Autodesk Inventor part; units mm, degrees
(part 2 of 2)
sketch "スケッチ16" plane through (250, 25, 10) normal (0, 1, 0) x (1, 0, 0)
  line L0 (-250, 20) -> (-250, 0) projected
  line L1 (-250, 0) -> (0, 0) projected
  line L2 (0, 0) -> (0, 20) projected
  line L3 (-250, 20) -> (0, 20) projected
  line L4 (-175, 16) -> (-158.2685, 16) projected
  line L5 (-158.2685, 16) -> (-175, 6.3111) projected
  line L6 (-175, 6.3111) -> (-175, 16) projected
  line L7 (-104, 13.8495) -> (-104, 4) projected
  line L8 (-104, 4) -> (-121.0089, 4) projected
  line L9 (-121.0089, 4) -> (-104, 13.8495) projected
  line L10 (-83, 16) -> (-72.9486, 16) projected
  line L11 (-72.9486, 16) -> (-83, 6.7218) projected
  line L12 (-83, 6.7218) -> (-83, 16) projected
  line L13 (-50, 16) -> (-43.9509, 16) projected
  line L14 (-43.9509, 16) -> (-50, 7.4601) projected
  line L15 (-50, 7.4601) -> (-50, 16) projected
  line L16 (-25, 16) -> (-18.9509, 16) projected
  line L17 (-18.9509, 16) -> (-25, 7.4601) projected
  line L18 (-25, 7.4601) -> (-25, 16) projected
  line L19 (-4, 4) -> (-10.0491, 4) projected
  line L20 (-10.0491, 4) -> (-4, 12.5399) projected
  line L21 (-4, 12.5399) -> (-4, 4) projected
  line L22 (-35.0491, 4) -> (-29, 12.5399) projected
  line L23 (-29, 12.5399) -> (-29, 4) projected
  line L24 (-29, 4) -> (-35.0491, 4) projected
  line L25 (-54, 4) -> (-63.1716, 4) projected
  line L26 (-63.1716, 4) -> (-54, 13.1716) projected
  line L27 (-54, 13.1716) -> (-54, 4) projected
  line L28 (-87, 4) -> (-97.0514, 4) projected
  line L29 (-97.0514, 4) -> (-87, 13.2782) projected
  line L30 (-87, 13.2782) -> (-87, 4) projected
  line L31 (-133.0311, 16) -> (-150, 6.3035) projected
  line L32 (-150, 6.3035) -> (-150, 16) projected
  line L33 (-150, 16) -> (-133.0311, 16) projected
  line L34 (-200, 16) -> (-183.0311, 16) projected
  line L35 (-183.0311, 16) -> (-200, 6.3035) projected
  line L36 (-200, 6.3035) -> (-200, 16) projected
  line L37 (-204, 4) -> (-240.5948, 4) projected
  line L38 (-240.5948, 4) -> (-204, 14.2649) projected
  line L39 (-204, 14.2649) -> (-204, 4) projected
  line L40 (-154, 13.8495) -> (-154, 4) projected
  line L41 (-154, 4) -> (-171.0089, 4) projected
  line L42 (-171.0089, 4) -> (-154, 13.8495) projected
  line L43 (-108.2685, 16) -> (-125, 6.3111) projected
  line L44 (-125, 6.3111) -> (-125, 16) projected
  line L45 (-125, 16) -> (-108.2685, 16) projected
  line L46 (-70, 4) -> (-80.0514, 4) projected
  line L47 (-80.0514, 4) -> (-70, 13.2782) projected
  line L48 (-70, 13.2782) -> (-70, 4) projected
  line L49 (-47.5491, 4) -> (-41.5, 12.5399) projected
  line L50 (-41.5, 12.5399) -> (-41.5, 4) projected
  line L51 (-41.5, 4) -> (-47.5491, 4) projected
  line L52 (-16.5, 4) -> (-22.5491, 4) projected
  line L53 (-22.5491, 4) -> (-16.5, 12.5399) projected
  line L54 (-16.5, 12.5399) -> (-16.5, 4) projected
  line L55 (-12.5, 16) -> (-6.4509, 16) projected
  line L56 (-6.4509, 16) -> (-12.5, 7.4601) projected
  line L57 (-12.5, 7.4601) -> (-12.5, 16) projected
  line L58 (-37.5, 16) -> (-31.4509, 16) projected
  line L59 (-31.4509, 16) -> (-37.5, 7.4601) projected
  line L60 (-37.5, 7.4601) -> (-37.5, 16) projected
  line L61 (-66, 16) -> (-56.8284, 16) projected
  line L62 (-56.8284, 16) -> (-66, 6.8284) projected
  line L63 (-66, 6.8284) -> (-66, 16) projected
  line L64 (-100, 16) -> (-89.9486, 16) projected
  line L65 (-89.9486, 16) -> (-100, 6.7218) projected
  line L66 (-100, 6.7218) -> (-100, 16) projected
  line L67 (-145.9689, 4) -> (-129, 13.6965) projected
  line L68 (-129, 13.6965) -> (-129, 4) projected
  line L69 (-129, 4) -> (-145.9689, 4) projected
  line L70 (-179, 13.6965) -> (-179, 4) projected
  line L71 (-179, 4) -> (-195.9689, 4) projected
  line L72 (-195.9689, 4) -> (-179, 13.6965) projected
  line L73 (-248, 16) -> (-211.4052, 16) projected
  line L74 (-211.4052, 16) -> (-248, 6.0772) projected
  line L75 (-248, 6.0772) -> (-248, 16) projected
  point P0 (-250, 10)
extrude "押し出し25" add sketch "スケッチ16" against normal blind 4 contours L13 L14 L15 | L25 L26 L27 | L49 L50 L51 | L61 L62 L63
extrude "押し出し26" cut sketch "スケッチ15" against normal blind 4 contours L11 L54 L109 L2 | L6 L41 L5 | L110 L104 L89 L14 | L12 L109 L54 | L41 L20 L19 L24 L5 | L89 L90 L15 L14 | L25 L7 L10 L9
sketch "スケッチ17" plane through (250, -25, -10) normal (0, -1, 0) x (1, 0, 0)
  line L0 (-31.0405, 4) -> (-25, 4) projected
  line L1 (-248, 13.9228) -> (-211.4052, 4) projected
  line L2 (-211.4052, 4) -> (-248, 4) projected
  line L3 (-248, 4) -> (-248, 13.9228) projected
  line L4 (-179, 16) -> (-179, 6.3035) projected
  line L5 (-179, 6.3035) -> (-195.9689, 16) projected
  line L6 (-195.9689, 16) -> (-179, 16) projected
  line L7 (-129, 6.3035) -> (-145.9689, 16) projected
  line L8 (-145.9689, 16) -> (-129, 16) projected
  line L9 (-129, 16) -> (-129, 6.3035) projected
  line L10 (-89.9486, 4) -> (-100, 4) projected
  line L11 (-100, 4) -> (-100, 13.2782) projected
  line L12 (-100, 13.2782) -> (-89.9486, 4) projected
  line L13 (-56.8284, 4) -> (-66, 4) projected
  line L14 (-66, 4) -> (-66, 13.1716) projected
  line L15 (-66, 13.1716) -> (-56.8284, 4) projected
  line L16 (-31.4509, 4) -> (-37.5, 4) projected
  line L17 (-37.5, 4) -> (-37.5, 12.5399) projected
  line L18 (-37.5, 12.5399) -> (-31.4509, 4) projected
  line L19 (-6.4509, 4) -> (-12.5, 4) projected
  line L20 (-12.5, 4) -> (-12.5, 12.5399) projected
  line L21 (-12.5, 12.5399) -> (-6.4509, 4) projected
  line L22 (-22.5491, 16) -> (-16.5, 16) projected
  line L23 (-16.5, 16) -> (-16.5, 7.4601) projected
  line L24 (-16.5, 7.4601) -> (-22.5491, 16) projected
  line L25 (-41.5, 7.4601) -> (-47.5491, 16) projected
  line L26 (-47.5491, 16) -> (-41.5, 16) projected
  line L27 (-41.5, 16) -> (-41.5, 7.4601) projected
  line L28 (-80.0514, 16) -> (-70, 16) projected
  line L29 (-70, 16) -> (-70, 6.7218) projected
  line L30 (-70, 6.7218) -> (-80.0514, 16) projected
  line L31 (-125, 13.6889) -> (-108.2685, 4) projected
  line L32 (-108.2685, 4) -> (-125, 4) projected
  line L33 (-125, 4) -> (-125, 13.6889) projected
  line L34 (-154, 16) -> (-154, 6.1505) projected
  line L35 (-154, 6.1505) -> (-171.0089, 16) projected
  line L36 (-171.0089, 16) -> (-154, 16) projected
  line L37 (-240.5948, 16) -> (-204, 16) projected
  line L38 (-204, 16) -> (-204, 5.7351) projected
  line L39 (-204, 5.7351) -> (-240.5948, 16) projected
  line L40 (-183.0311, 4) -> (-200, 4) projected
  line L41 (-200, 4) -> (-200, 13.6965) projected
  line L42 (-200, 13.6965) -> (-183.0311, 4) projected
  line L43 (-150, 13.6965) -> (-133.0311, 4) projected
  line L44 (-133.0311, 4) -> (-150, 4) projected
  line L45 (-150, 4) -> (-150, 13.6965) projected
  line L46 (-97.0514, 16) -> (-87, 16) projected
  line L47 (-87, 16) -> (-87, 6.7218) projected
  line L48 (-87, 6.7218) -> (-97.0514, 16) projected
  line L49 (-63.1716, 16) -> (-54, 16) projected
  line L50 (-54, 16) -> (-54, 6.8284) projected
  line L51 (-54, 6.8284) -> (-63.1716, 16) projected
  line L52 (-29, 7.4601) -> (-35.0491, 16) projected
  line L53 (-35.0491, 16) -> (-29, 16) projected
  line L54 (-29, 16) -> (-29, 7.4601) projected
  line L55 (-10.0491, 16) -> (-4, 16) projected
  line L56 (-4, 16) -> (-4, 7.4601) projected
  line L57 (-4, 7.4601) -> (-10.0491, 16) projected
  line L58 (-18.9509, 4) -> (-25, 4) projected
  line L59 (-25, 4) -> (-25, 12.5399) projected
  line L60 (-25, 12.5399) -> (-18.9509, 4) projected
  line L61 (-43.9509, 4) -> (-50, 4) projected
  line L62 (-50, 4) -> (-50, 12.5399) projected
  line L63 (-50, 12.5399) -> (-43.9509, 4) projected
  line L64 (-72.9486, 4) -> (-83, 4) projected
  line L65 (-83, 4) -> (-83, 13.2782) projected
  line L66 (-83, 13.2782) -> (-72.9486, 4) projected
  line L67 (-104, 16) -> (-104, 6.1505) projected
  line L68 (-104, 6.1505) -> (-121.0089, 16) projected
  line L69 (-121.0089, 16) -> (-104, 16) projected
  line L70 (-158.2685, 4) -> (-175, 4) projected
  line L71 (-175, 4) -> (-175, 13.6889) projected
  line L72 (-175, 13.6889) -> (-158.2685, 4) projected
  line L73 (-250, 20) -> (-250, 0) projected
  line L74 (-250, 0) -> (0, 0) projected
  line L75 (0, 0) -> (0, 20) projected
  line L76 (0, 20) -> (-250, 20) projected
  point P0 (-250, 10)
extrude "押し出し27" add sketch "スケッチ17" against normal blind 4 contours L13 L14 L15 | L25 L26 L27 | L49 L50 L51 | L61 L62 L63
mirror "ミラー4" about plane through (0, 0, 0) normal (0, 1, 0) of "押し出し26"
sketch "スケッチ18" plane through (250, -25, -10) normal (0, 0, -1) x (-1, 0, 0)
  line L0 (4, 46) -> (4, 50) projected
  line L1 (62.6667, 4) -> (50, 4) projected
  line L2 (4, 46) -> (52.1102, 46)
  line L3 (52.1102, 46) -> (52.1102, 4)
  line L4 (52.1102, 4) -> (4, 4)
  line L5 (4, 4) -> (4, 46)
  line L6 (53.3333, 4) -> (66, 4) projected
  line L7 (4, 46) -> (54, 46)
  line L8 (54, 46) -> (54, 4)
  line L9 (54, 4) -> (4, 4)
  line L10 (4, 4) -> (4, 46)
  point P0 (250, 25)
  dimension "d290" = 50
  constraints: 16 end point, 4 parallel, 2 horizontal, 2 perpendicular, 2 point on line
  measures "d290" distance of L8.end L9.end
extrude "押し出し28" add sketch "スケッチ18" against normal blind 4 contours L1 L4 L5 L2 L3
sketch "スケッチ19" plane through (250, -25, 10) normal (0, 0, 1) x (1, 0, 0)
  line L0 (-4, 4) -> (0, 4) projected
  line L1 (-50, 46) -> (-47.9595, 46) projected
  line L2 (-4, 4) -> (-47.9595, 4)
  line L3 (-47.9595, 4) -> (-47.9595, 46)
  line L4 (-47.9595, 46) -> (-4, 46)
  line L5 (-4, 46) -> (-4, 4)
  line L6 (-4, 4) -> (-54, 4)
  line L7 (-54, 4) -> (-54, 46)
  line L8 (-54, 46) -> (-4, 46)
  line L9 (-4, 46) -> (-4, 4)
  point P0 (-250, 25)
  dimension "d293" = 50
  dimension "d294" = 42
  constraints: 16 end point, 4 parallel, 2 horizontal, 2 perpendicular
  measures "d293" distance of L7.end L8.end
  measures "d294" distance of L6.end L7.end
extrude "押し出し29" add sketch "スケッチ19" against normal blind 4
sketch "スケッチ20" plane through (250, -25, -10) normal (0, 0, -1) x (-1, 0, 0)
  point P0 (250, 25)
extrude "押し出し30" add sketch "SCBottom" against normal blind 4 contours L99 L90 L43 L49 | L49 L43 L90 L101
sketch "スケッチ21" plane through (250, -25, 10) normal (0, 0, 1) x (1, 0, 0)
  line L0 (-54, 11.2801) -> (-57.92, 25) projected
  line L1 (-57.92, 25) -> (-54, 38.7199) projected
  line L2 (-54, 38.7199) -> (-54, 11.2801) projected
  line L3 (-250, 50) -> (-250, 0) projected
  line L4 (0, 0) -> (-250, 0) projected
  line L5 (0, 0) -> (0, 50) projected
  line L6 (-250, 50) -> (0, 50) projected
  line L7 (-248, 6.7649) -> (-248, 43.1716) projected
  line L8 (-248, 43.1716) -> (-229.3733, 24.5449) projected
  line L9 (-229.3733, 24.5449) -> (-248, 6.7649) projected
  line L10 (-197.7639, 46) -> (-181.2361, 46) projected
  line L11 (-181.2361, 46) -> (-189.5, 29.4721) projected
  line L12 (-189.5, 29.4721) -> (-197.7639, 46) projected
  line L13 (-162.2639, 25) -> (-154, 41.5279) projected
  line L14 (-154, 41.5279) -> (-154, 8.4721) projected
  line L15 (-154, 8.4721) -> (-162.2639, 25) projected
  line L16 (-129, 8.4721) -> (-137.2639, 25) projected
  line L17 (-137.2639, 25) -> (-129, 41.5279) projected
  line L18 (-129, 41.5279) -> (-129, 8.4721) projected
  line L19 (-104, 8.4721) -> (-112.2639, 25) projected
  line L20 (-112.2639, 25) -> (-104, 41.5279) projected
  line L21 (-104, 41.5279) -> (-104, 8.4721) projected
  line L22 (-87, 10.764) -> (-91.4064, 25) projected
  line L23 (-91.4064, 25) -> (-87, 39.236) projected
  line L24 (-87, 39.236) -> (-87, 10.764) projected
  line L25 (-74.4064, 25) -> (-70, 39.236) projected
  line L26 (-70, 39.236) -> (-70, 10.764) projected
  line L27 (-70, 10.764) -> (-74.4064, 25) projected
  line L28 (-63.92, 46) -> (-56.08, 46) projected
  line L29 (-56.08, 46) -> (-60, 32.2801) projected
  line L30 (-60, 32.2801) -> (-63.92, 46) projected
  line L31 (-72.0936, 4) -> (-80.9064, 4) projected
  line L32 (-80.9064, 4) -> (-76.5, 18.236) projected
  line L33 (-76.5, 18.236) -> (-72.0936, 4) projected
  line L34 (-89.0936, 4) -> (-97.9064, 4) projected
  line L35 (-97.9064, 4) -> (-93.5, 18.236) projected
  line L36 (-93.5, 18.236) -> (-89.0936, 4) projected
  line L37 (-122.7639, 46) -> (-106.2361, 46) projected
  line L38 (-106.2361, 46) -> (-114.5, 29.4721) projected
  line L39 (-114.5, 29.4721) -> (-122.7639, 46) projected
  line L40 (-131.2361, 4) -> (-147.7639, 4) projected
  line L41 (-147.7639, 4) -> (-139.5, 20.5279) projected
  line L42 (-139.5, 20.5279) -> (-131.2361, 4) projected
  line L43 (-156.2361, 4) -> (-172.7639, 4) projected
  line L44 (-172.7639, 4) -> (-164.5, 20.5279) projected
  line L45 (-164.5, 20.5279) -> (-156.2361, 4) projected
  line L46 (-187.2639, 25) -> (-179, 41.5279) projected
  line L47 (-179, 41.5279) -> (-179, 8.4721) projected
  line L48 (-179, 8.4721) -> (-187.2639, 25) projected
  line L49 (-191.7361, 25) -> (-200, 8.4721) projected
  line L50 (-200, 8.4721) -> (-200, 41.5279) projected
  line L51 (-200, 41.5279) -> (-191.7361, 25) projected
  line L52 (-172.7639, 46) -> (-156.2361, 46) projected
  line L53 (-156.2361, 46) -> (-164.5, 29.4721) projected
  line L54 (-164.5, 29.4721) -> (-172.7639, 46) projected
  line L55 (-150, 41.5279) -> (-141.7361, 25) projected
  line L56 (-141.7361, 25) -> (-150, 8.4721) projected
  line L57 (-150, 8.4721) -> (-150, 41.5279) projected
  line L58 (-106.2361, 4) -> (-122.7639, 4) projected
  line L59 (-122.7639, 4) -> (-114.5, 20.5279) projected
  line L60 (-114.5, 20.5279) -> (-106.2361, 4) projected
  line L61 (-97.9064, 46) -> (-89.0936, 46) projected
  line L62 (-89.0936, 46) -> (-93.5, 31.764) projected
  line L63 (-93.5, 31.764) -> (-97.9064, 46) projected
  line L64 (-80.9064, 46) -> (-72.0936, 46) projected
  line L65 (-72.0936, 46) -> (-76.5, 31.764) projected
  line L66 (-76.5, 31.764) -> (-80.9064, 46) projected
  line L67 (-56.08, 4) -> (-63.92, 4) projected
  line L68 (-63.92, 4) -> (-60, 17.7199) projected
  line L69 (-60, 17.7199) -> (-56.08, 4) projected
  line L70 (-62.08, 25) -> (-66, 11.2801) projected
  line L71 (-66, 11.2801) -> (-66, 38.7199) projected
  line L72 (-66, 38.7199) -> (-62.08, 25) projected
  line L73 (-78.5936, 25) -> (-83, 10.764) projected
  line L74 (-83, 10.764) -> (-83, 39.236) projected
  line L75 (-83, 39.236) -> (-78.5936, 25) projected
  line L76 (-95.5936, 25) -> (-100, 10.764) projected
  line L77 (-100, 10.764) -> (-100, 39.236) projected
  line L78 (-100, 39.236) -> (-95.5936, 25) projected
  line L79 (-125, 41.5279) -> (-116.7361, 25) projected
  line L80 (-116.7361, 25) -> (-125, 8.4721) projected
  line L81 (-125, 8.4721) -> (-125, 41.5279) projected
  line L82 (-147.7639, 46) -> (-131.2361, 46) projected
  line L83 (-131.2361, 46) -> (-139.5, 29.4721) projected
  line L84 (-139.5, 29.4721) -> (-147.7639, 46) projected
  line L85 (-166.7361, 25) -> (-175, 8.4721) projected
  line L86 (-175, 8.4721) -> (-175, 41.5279) projected
  line L87 (-175, 41.5279) -> (-166.7361, 25) projected
  line L88 (-197.7639, 4) -> (-189.5, 20.5279) projected
  line L89 (-189.5, 20.5279) -> (-181.2361, 4) projected
  line L90 (-181.2361, 4) -> (-197.7639, 4) projected
  line L91 (-226.4791, 27.3075) -> (-245.1716, 46) projected
  line L92 (-245.1716, 46) -> (-206.8966, 46) projected
  line L93 (-206.8966, 46) -> (-226.4791, 27.3075) projected
  line L94 (-245.1034, 4) -> (-226.5441, 21.7157) projected
  line L95 (-226.5441, 21.7157) -> (-208.8284, 4) projected
  line L96 (-208.8284, 4) -> (-245.1034, 4) projected
  line L97 (-204, 43.2351) -> (-204, 4.8284) projected
  line L98 (-204, 4.8284) -> (-223.6499, 24.4784) projected
  line L99 (-223.6499, 24.4784) -> (-204, 43.2351) projected
  point P0 (-250, 25)
extrude "押し出し31" add sketch "スケッチ21" against normal blind 4 contours L0 L1 L2
sketch "スケッチ22" plane through (250, -25, 10) normal (0, 0, 1) x (1, 0, 0)
  line L0 (-250, 50) -> (-250, 0) projected
  line L1 (0, 0) -> (-250, 0) projected
  line L2 (0, 0) -> (0, 50) projected
  line L3 (-250, 50) -> (0, 50) projected
  line L4 (-248, 6.7649) -> (-248, 43.1716) projected
  line L5 (-248, 43.1716) -> (-229.3733, 24.5449) projected
  line L6 (-229.3733, 24.5449) -> (-248, 6.7649) projected
  line L7 (-197.7639, 46) -> (-181.2361, 46) projected
  line L8 (-181.2361, 46) -> (-189.5, 29.4721) projected
  line L9 (-189.5, 29.4721) -> (-197.7639, 46) projected
  line L10 (-162.2639, 25) -> (-154, 41.5279) projected
  line L11 (-154, 41.5279) -> (-154, 8.4721) projected
  line L12 (-154, 8.4721) -> (-162.2639, 25) projected
  line L13 (-129, 8.4721) -> (-137.2639, 25) projected
  line L14 (-137.2639, 25) -> (-129, 41.5279) projected
  line L15 (-129, 41.5279) -> (-129, 8.4721) projected
  line L16 (-104, 8.4721) -> (-112.2639, 25) projected
  line L17 (-112.2639, 25) -> (-104, 41.5279) projected
  line L18 (-104, 41.5279) -> (-104, 8.4721) projected
  line L19 (-87, 10.764) -> (-91.4064, 25) projected
  line L20 (-91.4064, 25) -> (-87, 39.236) projected
  line L21 (-87, 39.236) -> (-87, 10.764) projected
  line L22 (-74.4064, 25) -> (-70, 39.236) projected
  line L23 (-70, 39.236) -> (-70, 10.764) projected
  line L24 (-70, 10.764) -> (-74.4064, 25) projected
  line L25 (-63.92, 46) -> (-56.08, 46) projected
  line L26 (-56.08, 46) -> (-60, 32.2801) projected
  line L27 (-60, 32.2801) -> (-63.92, 46) projected
  line L28 (-72.0936, 4) -> (-80.9064, 4) projected
  line L29 (-80.9064, 4) -> (-76.5, 18.236) projected
  line L30 (-76.5, 18.236) -> (-72.0936, 4) projected
  line L31 (-89.0936, 4) -> (-97.9064, 4) projected
  line L32 (-97.9064, 4) -> (-93.5, 18.236) projected
  line L33 (-93.5, 18.236) -> (-89.0936, 4) projected
  line L34 (-122.7639, 46) -> (-106.2361, 46) projected
  line L35 (-106.2361, 46) -> (-114.5, 29.4721) projected
  line L36 (-114.5, 29.4721) -> (-122.7639, 46) projected
  line L37 (-131.2361, 4) -> (-147.7639, 4) projected
  line L38 (-147.7639, 4) -> (-139.5, 20.5279) projected
  line L39 (-139.5, 20.5279) -> (-131.2361, 4) projected
  line L40 (-156.2361, 4) -> (-172.7639, 4) projected
  line L41 (-172.7639, 4) -> (-164.5, 20.5279) projected
  line L42 (-164.5, 20.5279) -> (-156.2361, 4) projected
  line L43 (-187.2639, 25) -> (-179, 41.5279) projected
  line L44 (-179, 41.5279) -> (-179, 8.4721) projected
  line L45 (-179, 8.4721) -> (-187.2639, 25) projected
  line L46 (-191.7361, 25) -> (-200, 8.4721) projected
  line L47 (-200, 8.4721) -> (-200, 41.5279) projected
  line L48 (-200, 41.5279) -> (-191.7361, 25) projected
  line L49 (-172.7639, 46) -> (-156.2361, 46) projected
  line L50 (-156.2361, 46) -> (-164.5, 29.4721) projected
  line L51 (-164.5, 29.4721) -> (-172.7639, 46) projected
  line L52 (-150, 41.5279) -> (-141.7361, 25) projected
  line L53 (-141.7361, 25) -> (-150, 8.4721) projected
  line L54 (-150, 8.4721) -> (-150, 41.5279) projected
  line L55 (-106.2361, 4) -> (-122.7639, 4) projected
  line L56 (-122.7639, 4) -> (-114.5, 20.5279) projected
  line L57 (-114.5, 20.5279) -> (-106.2361, 4) projected
  line L58 (-97.9064, 46) -> (-89.0936, 46) projected
  line L59 (-89.0936, 46) -> (-93.5, 31.764) projected
  line L60 (-93.5, 31.764) -> (-97.9064, 46) projected
  line L61 (-80.9064, 46) -> (-72.0936, 46) projected
  line L62 (-72.0936, 46) -> (-76.5, 31.764) projected
  line L63 (-76.5, 31.764) -> (-80.9064, 46) projected
  line L64 (-56.08, 4) -> (-63.92, 4) projected
  line L65 (-63.92, 4) -> (-60, 17.7199) projected
  line L66 (-60, 17.7199) -> (-56.08, 4) projected
  line L67 (-62.08, 25) -> (-66, 11.2801) projected
  line L68 (-66, 11.2801) -> (-66, 38.7199) projected
  line L69 (-66, 38.7199) -> (-62.08, 25) projected
  line L70 (-78.5936, 25) -> (-83, 10.764) projected
  line L71 (-83, 10.764) -> (-83, 39.236) projected
  line L72 (-83, 39.236) -> (-78.5936, 25) projected
  line L73 (-95.5936, 25) -> (-100, 10.764) projected
  line L74 (-100, 10.764) -> (-100, 39.236) projected
  line L75 (-100, 39.236) -> (-95.5936, 25) projected
  line L76 (-125, 41.5279) -> (-116.7361, 25) projected
  line L77 (-116.7361, 25) -> (-125, 8.4721) projected
  line L78 (-125, 8.4721) -> (-125, 41.5279) projected
  line L79 (-147.7639, 46) -> (-131.2361, 46) projected
  line L80 (-131.2361, 46) -> (-139.5, 29.4721) projected
  line L81 (-139.5, 29.4721) -> (-147.7639, 46) projected
  line L82 (-166.7361, 25) -> (-175, 8.4721) projected
  line L83 (-175, 8.4721) -> (-175, 41.5279) projected
  line L84 (-175, 41.5279) -> (-166.7361, 25) projected
  line L85 (-197.7639, 4) -> (-189.5, 20.5279) projected
  line L86 (-189.5, 20.5279) -> (-181.2361, 4) projected
  line L87 (-181.2361, 4) -> (-197.7639, 4) projected
  line L88 (-226.4791, 27.3075) -> (-245.1716, 46) projected
  line L89 (-245.1716, 46) -> (-206.8966, 46) projected
  line L90 (-206.8966, 46) -> (-226.4791, 27.3075) projected
  line L91 (-245.1034, 4) -> (-226.5441, 21.7157) projected
  line L92 (-226.5441, 21.7157) -> (-208.8284, 4) projected
  line L93 (-208.8284, 4) -> (-245.1034, 4) projected
  line L94 (-204, 43.2351) -> (-204, 4.8284) projected
  line L95 (-204, 4.8284) -> (-223.6499, 24.4784) projected
  line L96 (-223.6499, 24.4784) -> (-204, 43.2351) projected
  line L97 (-58.279, 25) -> (-48.0006, 4)
  line L98 (-50, 4) -> (-43.864, 4) projected
  line L99 (-58.279, 25) -> (-48.0006, 46)
  line L100 (-50, 46) -> (-43.864, 46) projected
  line L101 (-63.92, 46) -> (-60, 32.2801) projected
  line L102 (-60, 32.2801) -> (-53.2848, 46)
  line L103 (-53.3333, 46) -> (-46, 46) projected
  line L104 (-50, 4) -> (-46, 4)
  line L105 (-46, 4) -> (-46, 46)
  line L106 (-46, 46) -> (-50, 46)
  line L107 (-50, 46) -> (-50, 4)
  line L108 (-3.6692, 25) -> (16.3308, 25)
  line L109 (0, 46) -> (0, 4) projected
  line L110 (-3.6692, 25) -> (16.3308, 25) construction
  line L111 (-16.5, 4) -> (-10.0491, 4) projected
  line L112 (-15.3736, 4) -> (-19.3736, 4)
  line L113 (-19.3736, 4) -> (-19.3736, 46)
  line L114 (-19.3736, 46) -> (-15.3736, 46)
  line L115 (-15.3736, 46) -> (-15.3736, 4)
  line L116 (-30.6182, 3.9696) -> (-34.6182, 3.9696)
  line L117 (-34.6182, 3.9696) -> (-34.6182, 45.9696)
  line L118 (-34.6182, 45.9696) -> (-30.6182, 45.9696)
  line L119 (-30.6182, 45.9696) -> (-30.6182, 3.9696)
  line L120 (-4, 4) -> (0, 4) projected
  line L121 (-4, 4) -> (-15.3736, 46)
  line L122 (-30.6182, 45.9696) -> (-19.3736, 4)
  line L123 (-34.6182, 3.9696) -> (-46, 46)
  line L124 (-36.5487, 3.4469) -> (-47.9305, 45.4772)
  line L125 (-34.6182, 11.6212) -> (-44.0695, 46.5228)
  line L126 (-32.5501, 45.4521) -> (-21.3054, 3.4824)
  line L127 (-15.3736, 38.3484) -> (-6.0638, 3.9696)
  line L128 (-5.5304, 2) -> (0, 2)
  line L129 (-13.3015, 46) -> (-2.4696, 6)
  line L130 (-2.4696, 6) -> (0, 6)
  line L131 (-28.6863, 46.4872) -> (-19.3736, 11.7281)
  line L132 (-250, 50) -> (-250, 0) projected
  line L133 (0, 0) -> (-250, 0) projected
  line L134 (0, 0) -> (0, 50) projected
  line L135 (-250, 50) -> (0, 50) projected
  line L136 (-248, 6.7649) -> (-248, 43.1716) projected
  line L137 (-248, 43.1716) -> (-229.3733, 24.5449) projected
  line L138 (-229.3733, 24.5449) -> (-248, 6.7649) projected
  line L139 (-197.7639, 46) -> (-181.2361, 46) projected
  line L140 (-181.2361, 46) -> (-189.5, 29.4721) projected
  line L141 (-189.5, 29.4721) -> (-197.7639, 46) projected
  line L142 (-162.2639, 25) -> (-154, 41.5279) projected
  line L143 (-154, 41.5279) -> (-154, 8.4721) projected
  line L144 (-154, 8.4721) -> (-162.2639, 25) projected
  line L145 (-129, 8.4721) -> (-137.2639, 25) projected
  line L146 (-137.2639, 25) -> (-129, 41.5279) projected
  line L147 (-129, 41.5279) -> (-129, 8.4721) projected
  line L148 (-104, 8.4721) -> (-112.2639, 25) projected
  line L149 (-112.2639, 25) -> (-104, 41.5279) projected
  line L150 (-104, 41.5279) -> (-104, 8.4721) projected
  line L151 (-87, 10.764) -> (-91.4064, 25) projected
  line L152 (-91.4064, 25) -> (-87, 39.236) projected
  line L153 (-87, 39.236) -> (-87, 10.764) projected
  line L154 (-74.4064, 25) -> (-70, 39.236) projected
  line L155 (-70, 39.236) -> (-70, 10.764) projected
  line L156 (-70, 10.764) -> (-74.4064, 25) projected
  line L157 (-63.92, 46) -> (-56.08, 46) projected
  line L158 (-56.08, 46) -> (-60, 32.2801) projected
  line L159 (-60, 32.2801) -> (-63.92, 46) projected
  line L160 (-72.0936, 4) -> (-80.9064, 4) projected
  line L161 (-80.9064, 4) -> (-76.5, 18.236) projected
  line L162 (-76.5, 18.236) -> (-72.0936, 4) projected
  line L163 (-89.0936, 4) -> (-97.9064, 4) projected
  line L164 (-97.9064, 4) -> (-93.5, 18.236) projected
  line L165 (-93.5, 18.236) -> (-89.0936, 4) projected
  line L166 (-122.7639, 46) -> (-106.2361, 46) projected
  line L167 (-106.2361, 46) -> (-114.5, 29.4721) projected
  line L168 (-114.5, 29.4721) -> (-122.7639, 46) projected
  line L169 (-131.2361, 4) -> (-147.7639, 4) projected
  line L170 (-147.7639, 4) -> (-139.5, 20.5279) projected
  line L171 (-139.5, 20.5279) -> (-131.2361, 4) projected
  line L172 (-156.2361, 4) -> (-172.7639, 4) projected
  line L173 (-172.7639, 4) -> (-164.5, 20.5279) projected
  line L174 (-164.5, 20.5279) -> (-156.2361, 4) projected
  line L175 (-187.2639, 25) -> (-179, 41.5279) projected
  line L176 (-179, 41.5279) -> (-179, 8.4721) projected
  line L177 (-179, 8.4721) -> (-187.2639, 25) projected
  line L178 (-191.7361, 25) -> (-200, 8.4721) projected
  line L179 (-200, 8.4721) -> (-200, 41.5279) projected
  line L180 (-200, 41.5279) -> (-191.7361, 25) projected
  line L181 (-172.7639, 46) -> (-156.2361, 46) projected
  line L182 (-156.2361, 46) -> (-164.5, 29.4721) projected
  line L183 (-164.5, 29.4721) -> (-172.7639, 46) projected
  line L184 (-150, 41.5279) -> (-141.7361, 25) projected
  line L185 (-141.7361, 25) -> (-150, 8.4721) projected
  line L186 (-150, 8.4721) -> (-150, 41.5279) projected
  line L187 (-106.2361, 4) -> (-122.7639, 4) projected
  line L188 (-122.7639, 4) -> (-114.5, 20.5279) projected
  line L189 (-114.5, 20.5279) -> (-106.2361, 4) projected
  line L190 (-97.9064, 46) -> (-89.0936, 46) projected
  line L191 (-89.0936, 46) -> (-93.5, 31.764) projected
  line L192 (-93.5, 31.764) -> (-97.9064, 46) projected
  line L193 (-80.9064, 46) -> (-72.0936, 46) projected
  line L194 (-72.0936, 46) -> (-76.5, 31.764) projected
  line L195 (-76.5, 31.764) -> (-80.9064, 46) projected
  line L196 (-56.08, 4) -> (-63.92, 4) projected
  line L197 (-63.92, 4) -> (-60, 17.7199) projected
  line L198 (-60, 17.7199) -> (-56.08, 4) projected
  line L199 (-62.08, 25) -> (-66, 11.2801) projected
  line L200 (-66, 11.2801) -> (-66, 38.7199) projected
  line L201 (-66, 38.7199) -> (-62.08, 25) projected
  line L202 (-78.5936, 25) -> (-83, 10.764) projected
  line L203 (-83, 10.764) -> (-83, 39.236) projected
  line L204 (-83, 39.236) -> (-78.5936, 25) projected
  line L205 (-95.5936, 25) -> (-100, 10.764) projected
  line L206 (-100, 10.764) -> (-100, 39.236) projected
  line L207 (-100, 39.236) -> (-95.5936, 25) projected
  line L208 (-125, 41.5279) -> (-116.7361, 25) projected
  line L209 (-116.7361, 25) -> (-125, 8.4721) projected
  line L210 (-125, 8.4721) -> (-125, 41.5279) projected
  line L211 (-147.7639, 46) -> (-131.2361, 46) projected
  line L212 (-131.2361, 46) -> (-139.5, 29.4721) projected
  line L213 (-139.5, 29.4721) -> (-147.7639, 46) projected
  line L214 (-166.7361, 25) -> (-175, 8.4721) projected
  line L215 (-175, 8.4721) -> (-175, 41.5279) projected
  line L216 (-175, 41.5279) -> (-166.7361, 25) projected
  line L217 (-197.7639, 4) -> (-189.5, 20.5279) projected
  line L218 (-189.5, 20.5279) -> (-181.2361, 4) projected
  line L219 (-181.2361, 4) -> (-197.7639, 4) projected
  line L220 (-226.4791, 27.3075) -> (-245.1716, 46) projected
  line L221 (-245.1716, 46) -> (-206.8966, 46) projected
  line L222 (-206.8966, 46) -> (-226.4791, 27.3075) projected
  line L223 (-245.1034, 4) -> (-226.5441, 21.7157) projected
  line L224 (-226.5441, 21.7157) -> (-208.8284, 4) projected
  line L225 (-208.8284, 4) -> (-245.1034, 4) projected
  line L226 (-204, 43.2351) -> (-204, 4.8284) projected
  line L227 (-204, 4.8284) -> (-223.6499, 24.4784) projected
  line L228 (-223.6499, 24.4784) -> (-204, 43.2351) projected
  line L229 (-36.5487, 46.5531) -> (-47.9305, 4.5228)
  line L230 (-34.6182, 38.3788) -> (-44.0695, 3.4772)
  line L231 (-32.5501, 4.5479) -> (-21.3054, 46.5176)
  line L232 (-15.3736, 11.6516) -> (-6.0638, 46.0304)
  line L233 (-13.3015, 4) -> (-2.4696, 44)
  line L234 (-28.6863, 3.5128) -> (-19.3736, 38.2719)
  line L235 (-4, 11.6516) -> (-4, 38.3484)
  line L236 (-7.6148, 25) -> (-4, 38.3484)
  line L237 (-4, 11.6516) -> (-7.6148, 25)
  line L238 (-9.6868, 32.6516) -> (-6.0638, 46.0304)
  line L239 (-13.3015, 46) -> (-9.6868, 32.6516)
  line L240 (-11.7588, 25) -> (-15.3736, 11.6516)
  line L241 (-15.3736, 38.3484) -> (-11.7588, 25)
  line L242 (-9.6868, 17.3484) -> (-13.3015, 4)
  line L243 (-4, 11.6516) -> (-7.6148, 25)
  line L244 (-4, 38.3484) -> (-7.6148, 25)
  line L245 (-4, 11.6516) -> (-4, 38.3484)
  point P0 (-250, 25)
  point P1 (-50, 8.085)
  point P2 (-50, 41.915)
  point P3 (-46, 11.6516)
  point P4 (-42.3852, 25)
  point P5 (-46, 38.3484)
  dimension "d301" = 20
  dimension "d302" = 0
  dimension "d303" = 25
  dimension "d304" = 4
  dimension "d305" = 4
  dimension "d306" = 2
  dimension "d307" = 4
  dimension "d308" = 2
  dimension "d310" = 2
  dimension "d311" = 4
  dimension "d312" = 4
  constraints: 90 end point, 20 point on line, 13 parallel, 12 symmetric about line, 9 collinear, 4 horizontal, 4 perpendicular, 1 vertical
  measures "d301" distance of L108.start L108.end
  measures "d302" distance between parallel lines of L108 L110
  measures "d303" distance between parallel lines of L1 L108
  measures "d304" distance of L113.end L114.end
  measures "d305" distance of L117.end L118.end
  measures "d306" distance between parallel lines of L123 L124
  measures "d307" distance between parallel lines of L124 L125
  measures "d308" distance between parallel lines of L122 L126
  measures "d310" distance between parallel lines of L121 L127
  measures "d311" distance between parallel lines of L127 L129
  measures "d312" distance between parallel lines of L126 L131
extrude "押し出し32" cut sketch "スケッチ22" against normal through all contours L229 L105 L124 | L107 L97 L99
extrude "押し出し33" add sketch "SCLeft" against normal blind 500 contours L7 L15 L20 L8 L23 L14 L9 L19 L22 L10 L21 L18
extrude "押し出し34" cut sketch "SCLeft" against normal blind 496 contours L7 L15 L20 L8 L23 L14 L9 L19 L22 L10 L21 L18
sketch "スケッチ24" plane through (250, -25, -10) normal (0, 0, -1) x (-1, 0, 0)
  line L0 (58.279, 25) -> (50, 8.085) projected
  line L1 (50, 8.085) -> (50, 41.915) projected
  line L2 (50, 41.915) -> (58.279, 25) projected
  line L3 (46, 38.3484) -> (46, 11.6516) projected
  line L4 (46, 11.6516) -> (42.3852, 25) projected
  line L5 (42.3852, 25) -> (46, 38.3484) projected
  line L6 (54.7947, 14.0615) -> (54, 11.2801) projected
  line L7 (54, 11.2801) -> (54, 12.4721) projected
  line L8 (54, 12.4721) -> (54.7947, 14.0615) projected
  line L9 (250, 0) -> (250, 50) projected
  line L10 (250, 50) -> (0, 50) projected
  line L11 (0, 50) -> (0, 0) projected
  line L12 (250, 0) -> (0, 0) projected
  line L13 (204, 43.2351) -> (223.6499, 24.4784) projected
  line L14 (223.6499, 24.4784) -> (204, 4.8284) projected
  line L15 (204, 4.8284) -> (204, 43.2351) projected
  line L16 (226.5441, 21.7157) -> (245.1034, 4) projected
  line L17 (245.1034, 4) -> (208.8284, 4) projected
  line L18 (208.8284, 4) -> (226.5441, 21.7157) projected
  line L19 (226.4791, 27.3075) -> (206.8966, 46) projected
  line L20 (206.8966, 46) -> (245.1716, 46) projected
  line L21 (245.1716, 46) -> (226.4791, 27.3075) projected
  line L22 (181.2361, 46) -> (197.7639, 46) projected
  line L23 (197.7639, 46) -> (189.5, 29.4721) projected
  line L24 (189.5, 29.4721) -> (181.2361, 46) projected
  line L25 (189.5, 20.5279) -> (197.7639, 4) projected
  line L26 (197.7639, 4) -> (181.2361, 4) projected
  line L27 (181.2361, 4) -> (189.5, 20.5279) projected
  line L28 (175, 41.5279) -> (175, 8.4721) projected
  line L29 (175, 8.4721) -> (166.7361, 25) projected
  line L30 (166.7361, 25) -> (175, 41.5279) projected
  line L31 (139.5, 29.4721) -> (131.2361, 46) projected
  line L32 (131.2361, 46) -> (147.7639, 46) projected
  line L33 (147.7639, 46) -> (139.5, 29.4721) projected
  line L34 (125, 8.4721) -> (116.7361, 25) projected
  line L35 (116.7361, 25) -> (125, 41.5279) projected
  line L36 (125, 41.5279) -> (125, 8.4721) projected
  line L37 (100, 39.236) -> (100, 10.764) projected
  line L38 (100, 10.764) -> (95.5936, 25) projected
  line L39 (95.5936, 25) -> (100, 39.236) projected
  line L40 (83, 39.236) -> (83, 10.764) projected
  line L41 (83, 10.764) -> (78.5936, 25) projected
  line L42 (78.5936, 25) -> (83, 39.236) projected
  line L43 (66, 38.7199) -> (66, 11.2801) projected
  line L44 (66, 11.2801) -> (62.08, 25) projected
  line L45 (62.08, 25) -> (66, 38.7199) projected
  line L46 (60, 17.7199) -> (63.92, 4) projected
  line L47 (63.92, 4) -> (56.08, 4) projected
  line L48 (56.08, 4) -> (60, 17.7199) projected
  line L49 (76.5, 31.764) -> (72.0936, 46) projected
  line L50 (72.0936, 46) -> (80.9064, 46) projected
  line L51 (80.9064, 46) -> (76.5, 31.764) projected
  line L52 (93.5, 31.764) -> (89.0936, 46) projected
  line L53 (89.0936, 46) -> (97.9064, 46) projected
  line L54 (97.9064, 46) -> (93.5, 31.764) projected
  line L55 (114.5, 20.5279) -> (122.7639, 4) projected
  line L56 (122.7639, 4) -> (106.2361, 4) projected
  line L57 (106.2361, 4) -> (114.5, 20.5279) projected
  line L58 (150, 8.4721) -> (141.7361, 25) projected
  line L59 (141.7361, 25) -> (150, 41.5279) projected
  line L60 (150, 41.5279) -> (150, 8.4721) projected
  line L61 (164.5, 29.4721) -> (156.2361, 46) projected
  line L62 (156.2361, 46) -> (172.7639, 46) projected
  line L63 (172.7639, 46) -> (164.5, 29.4721) projected
  line L64 (200, 41.5279) -> (200, 8.4721) projected
  line L65 (200, 8.4721) -> (191.7361, 25) projected
  line L66 (191.7361, 25) -> (200, 41.5279) projected
  line L67 (179, 8.4721) -> (179, 41.5279) projected
  line L68 (179, 41.5279) -> (187.2639, 25) projected
  line L69 (187.2639, 25) -> (179, 8.4721) projected
  line L70 (164.5, 20.5279) -> (172.7639, 4) projected
  line L71 (172.7639, 4) -> (156.2361, 4) projected
  line L72 (156.2361, 4) -> (164.5, 20.5279) projected
  line L73 (139.5, 20.5279) -> (147.7639, 4) projected
  line L74 (147.7639, 4) -> (131.2361, 4) projected
  line L75 (131.2361, 4) -> (139.5, 20.5279) projected
  line L76 (114.5, 29.4721) -> (106.2361, 46) projected
  line L77 (106.2361, 46) -> (122.7639, 46) projected
  line L78 (122.7639, 46) -> (114.5, 29.4721) projected
  line L79 (93.5, 18.236) -> (97.9064, 4) projected
  line L80 (97.9064, 4) -> (89.0936, 4) projected
  line L81 (89.0936, 4) -> (93.5, 18.236) projected
  line L82 (76.5, 18.236) -> (80.9064, 4) projected
  line L83 (80.9064, 4) -> (72.0936, 4) projected
  line L84 (72.0936, 4) -> (76.5, 18.236) projected
  line L85 (54.7947, 35.9385) -> (54, 37.5279) projected
  line L86 (54, 37.5279) -> (54, 38.7199) projected
  line L87 (54, 38.7199) -> (54.7947, 35.9385) projected
  line L88 (60, 32.2801) -> (56.08, 46) projected
  line L89 (56.08, 46) -> (63.92, 46) projected
  line L90 (63.92, 46) -> (60, 32.2801) projected
  line L91 (70, 10.764) -> (70, 39.236) projected
  line L92 (70, 39.236) -> (74.4064, 25) projected
  line L93 (74.4064, 25) -> (70, 10.764) projected
  line L94 (87, 39.236) -> (91.4064, 25) projected
  line L95 (91.4064, 25) -> (87, 10.764) projected
  line L96 (87, 10.764) -> (87, 39.236) projected
  line L97 (104, 41.5279) -> (112.2639, 25) projected
  line L98 (112.2639, 25) -> (104, 8.4721) projected
  line L99 (104, 8.4721) -> (104, 41.5279) projected
  line L100 (129, 41.5279) -> (137.2639, 25) projected
  line L101 (137.2639, 25) -> (129, 8.4721) projected
  line L102 (129, 8.4721) -> (129, 41.5279) projected
  line L103 (154, 41.5279) -> (162.2639, 25) projected
  line L104 (162.2639, 25) -> (154, 8.4721) projected
  line L105 (154, 8.4721) -> (154, 41.5279) projected
  line L106 (248, 6.7649) -> (229.3733, 24.5449) projected
  line L107 (229.3733, 24.5449) -> (248, 43.1716) projected
  line L108 (248, 43.1716) -> (248, 6.7649) projected
  line L109 (40.3852, 24.9682) -> (40.3852, 35.3062)
  line L110 (34.7705, 38.3484) -> (34.7705, 11.6516)
  line L111 (34.7705, 11.6516) -> (38.3852, 25)
  line L112 (38.3852, 25) -> (34.7705, 38.3484)
  line L113 (46, 11.6516) -> (42.3852, 25) projected
  line L114 (42.3852, 25) -> (46, 38.3484) projected
  line L115 (42.3852, 25) -> (46, 38.3484)
  line L116 (46, 38.3484) -> (46, 11.6516) projected
  line L117 (46, 38.3484) -> (46, 11.6516)
  line L118 (46, 11.6516) -> (42.3852, 25)
  line L119 (19.7705, 38.3484) -> (19.7705, 11.6516)
  line L120 (23.3852, 25) -> (19.7705, 38.3484)
  line L121 (27.3852, 25) -> (31, 38.3484)
  line L122 (31, 38.3484) -> (31, 11.6516)
  line L123 (31, 11.6516) -> (27.3852, 25)
  line L124 (19.7705, 11.6516) -> (23.3852, 25)
  line L125 (4.7705, 38.3484) -> (4.7705, 11.6516)
  line L126 (8.3852, 25) -> (4.7705, 38.3484)
  line L127 (12.3852, 25) -> (16, 38.3484)
  line L128 (16, 38.3484) -> (16, 11.6516)
  line L129 (16, 11.6516) -> (12.3852, 25)
  line L130 (4.7705, 11.6516) -> (8.3852, 25)
  point P0 (250, 25)
  dimension "d321" = 2
  dimension "d326" = 15
  constraints: 38 end point, 3 collinear, 3 symmetric about line, 1 horizontal, 1 vertical, 24 other
  measures "d321" distance from line of L4.end L109
  measures "d326" distance of L112.end L119.start
extrude "押し出し35" cut sketch "スケッチ24" against normal blind 496 contours L112 L111 L110
extrude "押し出し36" cut sketch "スケッチ24" against normal blind 496 contours L120 L124 L119 | L121 L122 L123 | L126 L130 L125 | L127 L128 L129
mirror "ミラー5" about plane through (0, 0, 0) normal (1, 0, 0)
